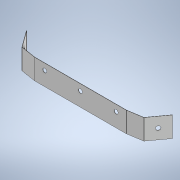
# Autodesk Inventor part: SIDE
Saved by Autodesk Inventor 2020 (Build 240168000, 168)
## iProperties
Created: 2022-07-14
Part Number: SIDE
Material: Generic
Document SubType Name: Sheet Metal
Designer: karimi2
Density: 1 g/cm^3
Sheet Metal Rule: Default_mm
Appearance: Default
Author: karimi2
Autodesk Inventor part; units mm, degrees
ref_plane "YZ Plane" through (0, 0, 0) normal (1, 0, 0) x (0, 1, 0)
ref_plane "XZ Plane" through (0, 0, 0) normal (0, 1, 0) x (-1, 0, 0)
ref_plane "XY Plane" through (0, 0, 0) normal (0, 0, 1) x (1, 0, 0)
sketch "Sketch1" plane through (0, 0, 0) normal (0, 0, 1) x (1, 0, 0)
  line L0 (0, 0) -> (-160, 0)
  line L1 (-160, 0) -> (-160, 40)
  line L2 (-160, 40) -> (0, 40)
  line L3 (0, 40) -> (0, 0) construction
  line L4 (0, 0) -> (160, 0)
  line L5 (160, 0) -> (160, 40)
  line L6 (160, 40) -> (0, 40)
  line L7 (-120, 40) -> (-120, 0)
  line L8 (120, 40) -> (120, 0)
  line L9 (90, 40) -> (90, 0)
  line L10 (-90, 40) -> (-90, 0)
  circle A0 centre (0, 27.5) radius 4
  circle A1 centre (70, 27.5) radius 4
  circle A2 centre (-70, 27.5) radius 4
  circle A3 centre (140, 20) radius 4
  circle A4 centre (-140, 20) radius 4
  dimension "d0" = 160
  dimension "d1" = 40
  dimension "d2" = 40
  dimension "d3" = 40
  dimension "d4" = 30
  dimension "d5" = 30
  dimension "d6" = 12.5
  dimension "d7" = 20
  dimension "d8" = 20
  dimension "d9" = 8
  dimension "d43" = 20
  dimension "d44" = 8
  dimension "d45" = 20
  dimension "d46" = 20
  constraints: 22 end point, 9 point on line, 5 centre point, 4 perpendicular, 3 equal radius, 3 horizontal alignment, 3 parallel, 2 symmetric about line, 1 horizontal
  measures "d0" distance of L1.end L2.end
  measures "d1" distance of L0.end L1.end
  measures "d2" distance from line of L0.end L7
  measures "d3" distance between parallel lines of L5 L8
  measures "d4" distance between parallel lines of L10 L7
  measures "d5" distance between parallel lines of L8 L9
  measures "d6" distance of L2.end A0.centre
  measures "d7" distance from line of L10 A2.centre
  measures "d8" distance from line of L9 A1.centre
  measures "d9" diameter of A0
  measures "d43" distance from line of L4 A3.centre
  measures "d44" diameter of A3
  measures "d45" distance from line of L1 A4.centre
  measures "d46" distance from line of L8 A3.centre
extrude "Plate2" add sketch "Sketch1" along normal blind 0.5
fold "Fold5" angle 45 bend radius 0.5 thickness 0.5 k factor 0.44 line from (120, 40, 0) to (120, 0, 0) line at bend centre moving side (1, 0, 0) folds toward (0, 0, -1)
fold "Fold6" angle 9 bend radius 0.5 thickness 0.5 k factor 0.44 line from (90, 40, 0) to (90, 0, 0) line at bend centre moving side (1, 0, 0) folds toward (0, 0, -1)
fold "Fold7" angle 45 bend radius 0.5 thickness 0.5 k factor 0.44 line from (-120, 40, 0) to (-120, 0, 0) line at bend centre moving side (-1, 0, 0) folds toward (0, 0, -1)
fold "Fold8" angle 9 bend radius 0.5 thickness 0.5 k factor 0.44 line from (-90, 40, 0) to (-90, 0, 0) line at bend centre moving side (-1, 0, 0) folds toward (0, 0, -1)
equation "\"d47\" = Thickness"
equation "\"d48\" = BendReliefWidth"
equation "\"d49\" = BendReliefDepth"
equation "\"d50\" = MinimumRemnant"
equation "\"d51\" = TransitionRadius"
equation "\"d53\" = BendRadius"
equation "\"d54\" = BendReliefWidth"
equation "\"d55\" = BendReliefDepth"
equation "\"d56\" = MinimumRemnant"
equation "\"d57\" = TransitionRadius"
equation "\"d59\" = BendRadius"
equation "\"d60\" = BendReliefWidth"
equation "\"d61\" = BendReliefDepth"
equation "\"d62\" = MinimumRemnant"
equation "\"d63\" = TransitionRadius"
equation "\"d65\" = BendRadius"
equation "\"d66\" = BendReliefWidth"
equation "\"d67\" = BendReliefDepth"
equation "\"d68\" = MinimumRemnant"
equation "\"d69\" = TransitionRadius"
equation "\"d71\" = BendRadius"
equation "\"BendRadius\" = Thickness"
equation "\"BendReliefWidth\" = Thickness"
equation "\"BendReliefDepth\" = 0.5 * Thickness"
equation "\"CornerReliefSize\" = 4 * Thickness"
equation "\"MinimumRemnant\" = 2 * Thickness"
equation "\"TransitionRadius\" = BendRadius"
equation "\"JacobiRadiusSize\" = BendRadius"
equation "\"GapSize\" = Thickness"
equation "\"Thickness\" = 0.5"
body "Solid2"
